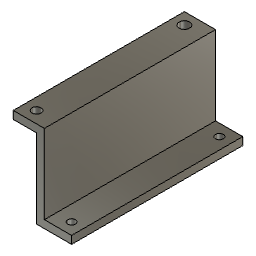
LidarMountLegs v1 (Autodesk Fusion 360 design; units mm, degrees)
Autodesk Fusion 360 part; units mm, degrees
sketch "Sketch1" plane through (0, 0, 0) normal (0, 0, 1) x (1, 0, 0)
  line L0 (-10, 72.4007) -> (12.5, 72.4007)
  line L1 (12.5, 72.4007) -> (12.5, -37.5993)
  line L2 (12.5, -37.5993) -> (-10, -37.5993)
  line L3 (-10, -37.5993) -> (-10, 72.4007)
  circle A0 centre (5, 64.9007) radius 2.5
  circle A1 centre (5, -30.0993) radius 2.5
  dimension "d1" = 5
  dimension "d2" = 5
  dimension "d3" = 95
  dimension "d4" = 15
  dimension "d5" = 7.5
  dimension "d6" = 7.5
  dimension "d7" = 7.5
  constraint horizontal L0
  constraint vertical L1
  constraint horizontal L2
  constraint vertical L3
  measures "d1" diameter of A0
  measures "d2" diameter of A1
  measures "d3" distance of A0.centre A1.centre
  measures "d4" distance of L3 A0.centre
  measures "d5" distance of L1 A0.centre
  measures "d6" distance of L0 A0.centre
  measures "d7" distance of L2 A1.centre
extrude "Extrude1" add sketch "Sketch1" along normal blind 5
sketch "Sketch2" plane through (0, 0, 5) normal (0, 0, 1) x (-1, 0, 0)
  circle A0 centre (-5, -64.9007) radius 2.5
  circle A1 centre (-5, 30.0993) radius 2.5
  line L0 (10, 37.5993) -> (-12.5, 37.5993)
  line L1 (-12.5, 37.5993) -> (-12.5, -72.4007)
  line L2 (-12.5, -72.4007) -> (10, -72.4007)
  line L3 (10, -72.4007) -> (10, 37.5993)
  line L4 (10, -72.4007) -> (5, -72.4007)
  line L5 (5, -72.4007) -> (5, 37.5993)
  line L6 (5, 37.5993) -> (10, 37.5993)
  line L7 (10, 37.5993) -> (10, -72.4007)
  dimension "d10" = 5
  constraint horizontal L4
  constraint vertical L5
  constraint horizontal L6
  constraint vertical L7
  constraint coincident L0 L5.end
  constraint coincident L2.end L3.start
  measures "d10" distance of L5 L7
extrude "Extrude2" add sketch "Sketch2" along normal blind 50.8 contours L0 L2 L3 L4 L5 L6 L7
sketch "Sketch3" plane through (-10, 0, 0) normal (-1, 0, 0) x (0, -1, 0)
  line L0 (-72.4007, 0) -> (37.5993, 0)
  line L1 (37.5993, 0) -> (37.5993, 55.8)
  line L2 (37.5993, 55.8) -> (-72.4007, 55.8)
  line L3 (-72.4007, 55.8) -> (-72.4007, 0)
  line L4 (-72.4007, 55.8) -> (37.5993, 55.8)
  line L5 (37.5993, 55.8) -> (37.5993, 50.8)
  line L6 (37.5993, 50.8) -> (-72.4007, 50.8)
  line L7 (-72.4007, 50.8) -> (-72.4007, 55.8)
  dimension "d13" = 5
  constraint horizontal L4
  constraint vertical L5
  constraint horizontal L6
  constraint vertical L7
  constraint coincident L1 L5.end
  constraint coincident L2.end L3.start
  measures "d13" distance of L2.end L6.end
extrude "Extrude3" add sketch "Sketch3" along normal blind 15 contours L1 L2 L3 L4 L5 L6 L7
sketch "Sketch4" plane through (0, 0, 50.8) normal (0, 0, -1) x (1, 0, 0)
  line L0 (-10, -72.4007) -> (-10, 37.5993)
  line L1 (-10, 37.5993) -> (-25, 37.5993)
  line L2 (-25, 37.5993) -> (-25, -72.4007)
  line L3 (-25, -72.4007) -> (-10, -72.4007)
  circle A0 centre (-17.5, 30.0993) radius 2.8953
  circle A1 centre (-17.5, -64.9007) radius 3.4334
  dimension "d16" = 95
  dimension "d17" = 7.5
  dimension "d18" = 7.5
  measures "d16" distance of A0.centre A1.centre
  measures "d17" distance of L1 A0.centre
  measures "d18" distance of L2 A0.centre
extrude "Extrude4" cut sketch "Sketch4" against normal blind 20 contours A0 | A1
